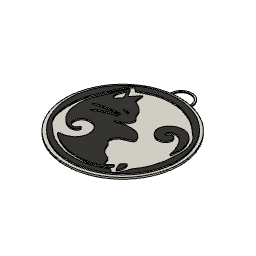
cats (Autodesk Fusion 360 design; units mm, degrees)
Autodesk Fusion 360 part; units mm, degrees
sketch "Sketch1" plane through (0, 0, 0) normal (0, 0, 1) x (1, 0, 0)
  spline S0 degree 3 poles (-11.5155, 73.2957) (-22.8925, 71.5759) (-32.7086, 67.8717) (-41.8102, 61.8657) knots 0 0 0 0 1 1 1 1
  spline S1 degree 3 poles (-41.8102, 61.8657) (-53.0815, 54.4309) (-62.9505, 42.6305) (-67.8452, 30.6977) knots 0 0 0 0 1 1 1 1
  spline S2 degree 3 poles (-67.8452, 30.6977) (-68.2421, 29.7452) (-68.7977, 28.4752) (-69.0623, 27.8667) knots 0 0 0 0 1 1 1 1
  spline S3 degree 3 poles (-69.0623, 27.8667) (-69.8561, 26.1469) (-71.9463, 18.9502) (-72.3696, 16.4632) knots 0 0 0 0 1 1 1 1
  spline S4 degree 3 poles (-72.3696, 16.4632) (-72.5813, 15.2461) (-72.8194, 14.1613) (-72.8723, 14.0555) knots 0 0 0 0 1 1 1 1
  spline S5 degree 3 poles (-72.8723, 14.0555) (-73.1634, 13.6057) (-73.8248, 4.5569) (-73.8248, 1.3025) knots 0 0 0 0 1 1 1 1
  spline S6 degree 3 poles (-73.8248, 1.3025) (-73.8248, -12.6939) (-69.1682, -26.955) (-60.4898, -39.4168) knots 0 0 0 0 1 1 1 1
  spline S7 degree 3 poles (-60.4898, -39.4168) (-58.4261, -42.4066) (-58.3732, -42.4595) (-54.96, -46.2431) knots 0 0 0 0 1 1 1 1
  spline S8 degree 3 poles (-54.96, -46.2431) (-51.0177, -50.6352) (-46.8373, -54.1541) (-41.2546, -57.8318) knots 0 0 0 0 1 1 1 1
  spline S9 degree 3 poles (-41.2546, -57.8318) (-37.8944, -60.0279) (-32.6292, -62.8325) (-29.3748, -64.1554) knots 0 0 0 0 1 1 1 1
  spline S10 degree 3 poles (-29.3748, -64.1554) (-28.4223, -64.5258) (-27.4169, -64.9491) (-27.1259, -65.0814) knots 0 0 0 0 1 1 1 1
  spline S11 degree 3 poles (-27.1259, -65.0814) (-25.9617, -65.5841) (-19.6117, -67.4627) (-18.0507, -67.7273) knots 0 0 0 0 1 1 1 1
  spline S12 degree 3 poles (-18.0507, -67.7273) (-17.1246, -67.886) (-16.0927, -68.1241) (-15.7752, -68.2564) knots 0 0 0 0 1 1 1 1
  spline S13 degree 3 poles (-15.7752, -68.2564) (-15.4577, -68.3623) (-13.7644, -68.6798) (-12.0182, -68.9708) knots 0 0 0 0 1 1 1 1
  spline S14 degree 3 poles (-12.0182, -68.9708) (-7.6261, -69.6323) (3.6716, -69.6323) (7.5345, -68.9443) knots 0 0 0 0 1 1 1 1
  spline S15 degree 3 poles (7.5345, -68.9443) (19.5202, -66.8277) (27.0873, -64.076) (35.7127, -58.7579) knots 0 0 0 0 1 1 1 1
  spline S16 degree 3 poles (35.7127, -58.7579) (48.201, -51.0056) (58.3081, -39.3375) (63.7585, -26.2935) knots 0 0 0 0 1 1 1 1
  spline S17 degree 3 poles (63.7585, -26.2935) (66.5631, -19.5995) (68.2035, -13.8052) (69.0502, -7.4023) knots 0 0 0 0 1 1 1 1
  spline S18 degree 3 poles (69.0502, -7.4023) (69.2089, -6.1587) (69.3941, -4.8623) (69.447, -4.4918) knots 0 0 0 0 1 1 1 1
  spline S19 degree 3 poles (69.447, -4.4918) (69.5264, -4.1214) (69.6323, -2.1106) (69.7381, 0.0061) knots 0 0 0 0 1 1 1 1
  spline S20 degree 3 poles (69.7381, 0.0061) (70.2143, 11.4096) (67.0923, 24.9298) (61.6154, 35.1427) knots 0 0 0 0 1 1 1 1
  spline S21 degree 3 poles (61.6154, 35.1427) (56.0327, 45.5673) (50.106, 52.5523) (40.8456, 59.6167) knots 0 0 0 0 1 1 1 1
  spline S22 degree 3 poles (40.8456, 59.6167) (31.3735, 66.8663) (19.0968, 71.814) (6.6614, 73.4015) knots 0 0 0 0 1 1 1 1
  spline S23 degree 3 poles (6.6614, 73.4015) (2.1106, 73.9836) (-7.2292, 73.9307) (-11.5155, 73.2957) knots 0 0 0 0 1 1 1 1
  spline S24 degree 3 poles (7.6668, 65.8609) (8.3283, 65.7286) (9.5718, 65.4905) (10.445, 65.3582) knots 0 0 0 0 1 1 1 1
  spline S25 degree 3 poles (10.445, 65.3582) (12.4293, 64.9877) (14.255, 64.4321) (20.2345, 62.2625) knots 0 0 0 0 1 1 1 1
  spline S26 degree 3 poles (20.2345, 62.2625) (26.1083, 60.1194) (28.0133, 59.2727) (31.982, 56.918) knots 0 0 0 0 1 1 1 1
  spline S27 degree 3 poles (31.982, 56.918) (36.427, 54.2986) (41.1631, 50.7002) (44.7085, 47.2607) knots 0 0 0 0 1 1 1 1
  spline S28 degree 3 poles (44.7085, 47.2607) (46.3754, 45.6467) (48.4656, 43.8475) (49.3387, 43.2655) knots 0 0 0 0 1 1 1 1
  spline S29 degree 3 poles (49.3387, 43.2655) (50.2118, 42.7098) (51.7993, 41.334) (52.8841, 40.2492) knots 0 0 0 0 1 1 1 1
  spline S30 degree 3 poles (52.8841, 40.2492) (54.8156, 38.2648) (58.4668, 33.423) (58.4668, 32.8409) knots 0 0 0 0 1 1 1 1
  spline S31 degree 3 poles (58.4668, 32.8409) (58.4668, 32.6821) (58.9431, 31.5973) (59.4987, 30.4596) knots 0 0 0 0 1 1 1 1
  spline S32 degree 3 poles (59.4987, 30.4596) (61.1391, 27.2052) (62.3033, 23.263) (62.9912, 18.6592) knots 0 0 0 0 1 1 1 1
  spline S33 degree 3 poles (62.9912, 18.6592) (63.3087, 16.3838) (63.15, 5.8798) (62.7002, 1.1173) knots 0 0 0 0 1 1 1 1
  spline S34 degree 3 poles (62.7002, 1.1173) (62.0387, -5.8148) (61.2714, -10.3656) (60.3454, -12.9585) knots 0 0 0 0 1 1 1 1
  spline S35 degree 3 poles (60.3454, -12.9585) (60.0014, -13.8845) (58.8373, -17.7475) (58.2287, -19.97) knots 0 0 0 0 1 1 1 1
  spline S36 degree 3 poles (58.2287, -19.97) (57.6202, -22.1925) (55.477, -27.0873) (54.1012, -29.4156) knots 0 0 0 0 1 1 1 1
  spline S37 degree 3 poles (54.1012, -29.4156) (53.5456, -30.3152) (52.0639, -32.617) (50.8468, -34.4691) knots 0 0 0 0 1 1 1 1
  spline S38 degree 3 poles (50.8468, -34.4691) (49.1006, -37.1414) (48.4656, -38.3585) (47.9893, -40.0254) knots 0 0 0 0 1 1 1 1
  spline S39 degree 3 poles (47.9893, -40.0254) (47.6454, -41.216) (47.3543, -42.3273) (47.3543, -42.5125) knots 0 0 0 0 1 1 1 1
  spline S40 degree 3 poles (47.3543, -42.5125) (47.3543, -43.1739) (45.2641, -47.6718) (44.2852, -49.1535) knots 0 0 0 0 1 1 1 1
  spline S41 degree 3 poles (44.2852, -49.1535) (41.9568, -52.6195) (40.8456, -53.8102) (39.5491, -54.3129) knots 0 0 0 0 1 1 1 1
  spline S42 degree 3 poles (39.5491, -54.3129) (38.0939, -54.842) (37.8823, -54.7362) (36.9827, -53.1223) knots 0 0 0 0 1 1 1 1
  spline S43 degree 3 poles (36.9827, -53.1223) (36.4006, -52.1168) (35.3687, -51.3231) (34.575, -51.3231) knots 0 0 0 0 1 1 1 1
  spline S44 degree 3 poles (34.575, -51.3231) (34.3898, -51.3231) (32.9345, -52.1698) (31.3206, -53.2281) knots 0 0 0 0 1 1 1 1
  spline S45 degree 3 poles (31.3206, -53.2281) (28.3043, -55.2125) (24.5737, -57.0645) (22.3512, -57.7525) knots 0 0 0 0 1 1 1 1
  spline S46 degree 3 poles (22.3512, -57.7525) (21.6368, -57.9641) (20.1023, -58.5198) (18.9645, -58.9695) knots 0 0 0 0 1 1 1 1
  spline S47 degree 3 poles (18.9645, -58.9695) (17.8268, -59.4193) (16.4775, -59.8956) (15.9218, -60.0279) knots 0 0 0 0 1 1 1 1
  spline S48 degree 3 poles (15.9218, -60.0279) (15.3927, -60.1602) (13.7523, -60.5835) (12.297, -60.9275) knots 0 0 0 0 1 1 1 1
  spline S49 degree 3 poles (12.297, -60.9275) (10.8418, -61.2979) (8.0373, -61.8535) (6.0793, -62.1975) knots 0 0 0 0 1 1 1 1
  spline S50 degree 3 poles (6.0793, -62.1975) (2.825, -62.7266) (1.9783, -62.7531) (-3.7102, -62.5943) knots 0 0 0 0 1 1 1 1
  spline S51 degree 3 poles (-3.7102, -62.5943) (-9.4517, -62.4356) (-13.8438, -62.0123) (-16.1457, -61.4037) knots 0 0 0 0 1 1 1 1
  spline S52 degree 3 poles (-16.1457, -61.4037) (-16.6484, -61.2714) (-17.7332, -60.9539) (-18.5269, -60.7158) knots 0 0 0 0 1 1 1 1
  spline S53 degree 3 poles (-18.5269, -60.7158) (-19.3207, -60.4777) (-21.0405, -60.0014) (-22.3634, -59.6575) knots 0 0 0 0 1 1 1 1
  spline S54 degree 3 poles (-22.3634, -59.6575) (-30.5655, -57.4614) (-40.7784, -51.9581) (-46.3082, -46.6929) knots 0 0 0 0 1 1 1 1
  spline S55 degree 3 poles (-46.3082, -46.6929) (-47.5517, -45.5287) (-49.9859, -43.412) (-51.7321, -42.0098) knots 0 0 0 0 1 1 1 1
  spline S56 degree 3 poles (-51.7321, -42.0098) (-55.0659, -39.3639) (-57.0502, -37.4589) (-58.5584, -35.4481) knots 0 0 0 0 1 1 1 1
  spline S57 degree 3 poles (-58.5584, -35.4481) (-59.9607, -33.596) (-62.8975, -28.2779) (-63.4796, -26.5581) knots 0 0 0 0 1 1 1 1
  spline S58 degree 3 poles (-63.4796, -26.5581) (-64.8025, -22.5629) (-65.8873, -17.7739) (-65.8873, -15.9748) knots 0 0 0 0 1 1 1 1
  spline S59 degree 3 poles (-65.8873, -15.9748) (-65.8873, -15.3398) (-66.0725, -13.9639) (-66.3107, -12.9056) knots 0 0 0 0 1 1 1 1
  spline S60 degree 3 poles (-66.3107, -12.9056) (-66.6546, -11.2916) (-66.7075, -9.8629) (-66.5752, -4.095) knots 0 0 0 0 1 1 1 1
  spline S61 degree 3 poles (-66.5752, -4.095) (-66.39, 3.1546) (-66.1255, 6.3825) (-65.5169, 8.9225) knots 0 0 0 0 1 1 1 1
  spline S62 degree 3 poles (-65.5169, 8.9225) (-65.3052, 9.7692) (-64.8819, 11.6477) (-64.5644, 13.103) knots 0 0 0 0 1 1 1 1
  spline S63 degree 3 poles (-64.5644, 13.103) (-64.2734, 14.5582) (-63.8765, 16.278) (-63.7177, 16.9394) knots 0 0 0 0 1 1 1 1
  spline S64 degree 3 poles (-63.7177, 16.9394) (-63.1886, 19.1619) (-58.9552, 29.5071) (-57.4471, 32.2852) knots 0 0 0 0 1 1 1 1
  spline S65 degree 3 poles (-57.4471, 32.2852) (-56.6005, 33.8198) (-55.7802, 35.619) (-55.6215, 36.3334) knots 0 0 0 0 1 1 1 1
  spline S66 degree 3 poles (-55.6215, 36.3334) (-55.4363, 37.0213) (-54.9865, 38.2648) (-54.6161, 39.1115) knots 0 0 0 0 1 1 1 1
  spline S67 degree 3 poles (-54.6161, 39.1115) (-54.2457, 39.9317) (-53.6371, 41.4663) (-53.2667, 42.4717) knots 0 0 0 0 1 1 1 1
  spline S68 degree 3 poles (-53.2667, 42.4717) (-52.473, 44.6942) (-49.3773, 51.1236) (-47.6046, 54.2457) knots 0 0 0 0 1 1 1 1
  spline S69 degree 3 poles (-47.6046, 54.2457) (-46.9167, 55.4892) (-45.7525, 57.0767) (-45.0117, 57.7911) knots 0 0 0 0 1 1 1 1
  line L0 (-45.0117, 57.7911) -> (-43.7152, 59.0875)
  line L1 (-43.7152, 59.0875) -> (-42.6834, 58.4525)
  spline S70 degree 3 poles (-42.6834, 58.4525) (-42.1277, 58.1086) (-41.043, 57.2619) (-40.3021, 56.5475) knots 0 0 0 0 1 1 1 1
  spline S71 degree 3 poles (-40.3021, 56.5475) (-39.0321, 55.3569) (-38.8205, 55.2511) (-37.9473, 55.3834) knots 0 0 0 0 1 1 1 1
  spline S72 degree 3 poles (-37.9473, 55.3834) (-37.4182, 55.4627) (-35.3015, 56.4946) (-33.2642, 57.6588) knots 0 0 0 0 1 1 1 1
  spline S73 degree 3 poles (-33.2642, 57.6588) (-31.2005, 58.823) (-28.978, 60.0136) (-28.3165, 60.3046) knots 0 0 0 0 1 1 1 1
  spline S74 degree 3 poles (-28.3165, 60.3046) (-22.0459, 63.0827) (-19.8498, 64.0352) (-19.5852, 64.0352) knots 0 0 0 0 1 1 1 1
  spline S75 degree 3 poles (-19.5852, 64.0352) (-19.4, 64.0352) (-18.2888, 64.2469) (-17.0982, 64.538) knots 0 0 0 0 1 1 1 1
  spline S76 degree 3 poles (-17.0982, 64.538) (-13.4734, 65.3846) (-10.2719, 65.9138) (-7.388, 66.1519) knots 0 0 0 0 1 1 1 1
  spline S77 degree 3 poles (-7.388, 66.1519) (-4.16, 66.4165) (5.947, 66.2313) (7.6668, 65.8609) knots 0 0 0 0 1 1 1 1
  spline S78 degree 3 poles (-29.6394, 52.0496) (-30.5919, 50.859) (-32.0207, 48.9805) (-32.8409, 47.8957) knots 0 0 0 0 1 1 1 1
  spline S79 degree 3 poles (-32.8409, 47.8957) (-33.6611, 46.8109) (-34.7459, 45.5144) (-35.2486, 45.0382) knots 0 0 0 0 1 1 1 1
  line L2 (-35.2486, 45.0382) -> (-36.2011, 44.1386)
  line L3 (-36.2011, 44.1386) -> (-37.3388, 44.5355)
  spline S80 degree 3 poles (-37.3388, 44.5355) (-38.3707, 44.8794) (-38.6617, 45.1705) (-39.773, 46.9961) knots 0 0 0 0 1 1 1 1
  spline S81 degree 3 poles (-39.773, 46.9961) (-40.4609, 48.1602) (-41.4663, 49.9594) (-42.0219, 51.0177) knots 0 0 0 0 1 1 1 1
  spline S82 degree 3 poles (-42.0219, 51.0177) (-43.3184, 53.5313) (-44.0857, 53.7959) (-45.0911, 52.0496) knots 0 0 0 0 1 1 1 1
  spline S83 degree 3 poles (-45.0911, 52.0496) (-45.9377, 50.568) (-47.8163, 46.7315) (-48.028, 46.0436) knots 0 0 0 0 1 1 1 1
  spline S84 degree 3 poles (-48.028, 46.0436) (-48.2132, 45.3821) (-48.7423, 44.165) (-49.88, 41.678) knots 0 0 0 0 1 1 1 1
  spline S85 degree 3 poles (-49.88, 41.678) (-50.4886, 40.3286) (-51.0971, 38.5294) (-52.129, 34.9311) knots 0 0 0 0 1 1 1 1
  spline S86 degree 3 poles (-52.129, 34.9311) (-52.4465, 33.8463) (-53.69, 30.9094) (-54.9071, 28.4488) knots 0 0 0 0 1 1 1 1
  spline S87 degree 3 poles (-54.9071, 28.4488) (-60.4369, 17.1775) (-62.2096, 9.3194) (-61.4688, -0.576) knots 0 0 0 0 1 1 1 1
  spline S88 degree 3 poles (-61.4688, -0.576) (-60.7015, -10.5243) (-57.8705, -17.8004) (-52.6846, -22.9598) knots 0 0 0 0 1 1 1 1
  spline S89 degree 3 poles (-52.6846, -22.9598) (-47.2871, -28.3573) (-43.8475, -30.1035) (-39.0586, -29.8125) knots 0 0 0 0 1 1 1 1
  spline S90 degree 3 poles (-39.0586, -29.8125) (-35.8042, -29.6273) (-34.349, -29.0452) (-33.0525, -27.4048) knots 0 0 0 0 1 1 1 1
  spline S91 degree 3 poles (-33.0525, -27.4048) (-31.8884, -25.976) (-31.6767, -25.3675) (-31.809, -24.0445) knots 0 0 0 0 1 1 1 1
  spline S92 degree 3 poles (-31.809, -24.0445) (-31.8619, -23.3831) (-32.1, -23.0391) (-32.735, -22.6952) knots 0 0 0 0 1 1 1 1
  line L4 (-32.735, -22.6952) -> (-33.5552, -22.1925)
  line L5 (-33.5552, -22.1925) -> (-35.0634, -24.2562)
  spline S93 degree 3 poles (-35.0634, -24.2562) (-36.9155, -26.7962) (-37.0477, -26.902) (-38.6088, -27.1137) knots 0 0 0 0 1 1 1 1
  spline S94 degree 3 poles (-38.6088, -27.1137) (-40.4873, -27.3783) (-42.4717, -26.4258) (-43.7682, -24.6266) knots 0 0 0 0 1 1 1 1
  spline S95 degree 3 poles (-43.7682, -24.6266) (-44.7207, -23.3302) (-44.7736, -23.1714) (-44.9059, -20.6579) knots 0 0 0 0 1 1 1 1
  spline S96 degree 3 poles (-44.9059, -20.6579) (-45.0911, -17.6152) (-44.7207, -16.1864) (-43.2919, -13.9375) knots 0 0 0 0 1 1 1 1
  spline S97 degree 3 poles (-43.2919, -13.9375) (-41.7838, -11.6356) (-40.5402, -10.8418) (-37.3123, -10.1539) knots 0 0 0 0 1 1 1 1
  spline S98 degree 3 poles (-37.3123, -10.1539) (-34.693, -9.6248) (-32.8673, -9.6248) (-30.4067, -10.1804) knots 0 0 0 0 1 1 1 1
  spline S99 degree 3 poles (-30.4067, -10.1804) (-27.655, -10.7889) (-26.2792, -11.5033) (-24.6388, -13.1437) knots 0 0 0 0 1 1 1 1
  spline S100 degree 3 poles (-24.6388, -13.1437) (-22.8132, -14.9958) (-21.8871, -16.5833) (-20.8817, -19.626) knots 0 0 0 0 1 1 1 1
  spline S101 degree 3 poles (-20.8817, -19.626) (-20.2202, -21.6368) (-20.1144, -22.3512) (-20.1144, -24.9177) knots 0 0 0 0 1 1 1 1
  spline S102 degree 3 poles (-20.1144, -24.9177) (-20.1144, -29.6537) (-21.1727, -32.4583) (-24.5859, -36.771) knots 0 0 0 0 1 1 1 1
  spline S103 degree 3 poles (-24.5859, -36.771) (-26.4644, -39.1523) (-27.5757, -39.9195) (-32.153, -42.0098) knots 0 0 0 0 1 1 1 1
  spline S104 degree 3 poles (-32.153, -42.0098) (-34.9311, -43.2798) (-35.2221, -43.3591) (-38.5823, -43.6766) knots 0 0 0 0 1 1 1 1
  spline S105 degree 3 poles (-38.5823, -43.6766) (-42.3923, -44.0206) (-42.3923, -44.0206) (-41.2017, -45.4758) knots 0 0 0 0 1 1 1 1
  spline S106 degree 3 poles (-41.2017, -45.4758) (-40.4609, -46.4283) (-34.058, -50.6881) (-31.5444, -51.9581) knots 0 0 0 0 1 1 1 1
  spline S107 degree 3 poles (-31.5444, -51.9581) (-29.0044, -53.2281) (-25.5384, -54.6568) (-22.9455, -55.4506) knots 0 0 0 0 1 1 1 1
  spline S108 degree 3 poles (-22.9455, -55.4506) (-21.8342, -55.7945) (-19.9292, -56.4031) (-18.7121, -56.7735) knots 0 0 0 0 1 1 1 1
  spline S109 degree 3 poles (-18.7121, -56.7735) (-13.3411, -58.4404) (-4.6363, -59.2341) (2.481, -58.7579) knots 0 0 0 0 1 1 1 1
  spline S110 degree 3 poles (2.481, -58.7579) (8.1166, -58.361) (11.3181, -57.7525) (15.7366, -56.2443) knots 0 0 0 0 1 1 1 1
  spline S111 degree 3 poles (15.7366, -56.2443) (22.2189, -54.0218) (25.8437, -52.355) (29.786, -49.7091) knots 0 0 0 0 1 1 1 1
  spline S112 degree 3 poles (29.786, -49.7091) (31.7968, -48.3598) (32.326, -47.8041) (33.1991, -46.2166) knots 0 0 0 0 1 1 1 1
  line L6 (33.1991, -46.2166) -> (33.7283, -45.2377)
  line L7 (33.7283, -45.2377) -> (32.9875, -44.5233)
  spline S113 degree 3 poles (32.9875, -44.5233) (32.4318, -43.9412) (32.1937, -43.8618) (32.035, -44.1264) knots 0 0 0 0 1 1 1 1
  spline S114 degree 3 poles (32.035, -44.1264) (31.9291, -44.3381) (30.8179, -45.5023) (29.6008, -46.7458) knots 0 0 0 0 1 1 1 1
  spline S115 degree 3 poles (29.6008, -46.7458) (27.3783, -48.9948) (25.6585, -50.1589) (24.9706, -49.8943) knots 0 0 0 0 1 1 1 1
  spline S116 degree 3 poles (24.9706, -49.8943) (24.3885, -49.6827) (23.6477, -47.9364) (22.9068, -44.9731) knots 0 0 0 0 1 1 1 1
  spline S117 degree 3 poles (22.9068, -44.9731) (22.0602, -41.7187) (21.3987, -40.8456) (19.0704, -39.9195) knots 0 0 0 0 1 1 1 1
  spline S118 degree 3 poles (19.0704, -39.9195) (15.0223, -38.332) (12.8791, -36.9827) (10.445, -34.5485) knots 0 0 0 0 1 1 1 1
  spline S119 degree 3 poles (10.445, -34.5485) (7.905, -31.982) (6.5291, -29.7595) (5.7089, -26.9814) knots 0 0 0 0 1 1 1 1
  spline S120 degree 3 poles (5.7089, -26.9814) (5.2062, -25.2352) (3.7775, -23.2508) (1.9518, -21.7691) knots 0 0 0 0 1 1 1 1
  spline S121 degree 3 poles (1.9518, -21.7691) (0.7348, -20.7902) (0.576, -20.5256) (0.4173, -19.335) knots 0 0 0 0 1 1 1 1
  spline S122 degree 3 poles (0.4173, -19.335) (0.1262, -17.0331) (1.1581, -14.1756) (3.3806, -11.2387) knots 0 0 0 0 1 1 1 1
  spline S123 degree 3 poles (3.3806, -11.2387) (4.5448, -9.7041) (5.4708, -9.122) (9.2543, -7.6404) knots 0 0 0 0 1 1 1 1
  spline S124 degree 3 poles (9.2543, -7.6404) (12.7998, -6.2381) (16.1864, -4.5712) (17.2183, -3.6981) knots 0 0 0 0 1 1 1 1
  spline S125 degree 3 poles (17.2183, -3.6981) (19.0968, -2.137) (18.1179, 1.4613) (14.9693, 4.6363) knots 0 0 0 0 1 1 1 1
  spline S126 degree 3 poles (14.9693, 4.6363) (12.2706, 7.335) (8.6987, 8.7373) (3.1689, 9.293) knots 0 0 0 0 1 1 1 1
  spline S127 degree 3 poles (3.1689, 9.293) (0.8141, 9.5311) (-0.6411, 9.5311) (-2.7048, 9.293) knots 0 0 0 0 1 1 1 1
  spline S128 degree 3 poles (-2.7048, 9.293) (-5.7211, 8.9755) (-6.9646, 8.6315) (-12.9177, 6.4355) knots 0 0 0 0 1 1 1 1
  spline S129 degree 3 poles (-12.9177, 6.4355) (-15.299, 5.5623) (-17.0452, 5.0596) (-17.1775, 5.1919) knots 0 0 0 0 1 1 1 1
  spline S130 degree 3 poles (-17.1775, 5.1919) (-17.3098, 5.3242) (-17.3627, 5.8005) (-17.2834, 6.2767) knots 0 0 0 0 1 1 1 1
  spline S131 degree 3 poles (-17.2834, 6.2767) (-17.0982, 7.388) (-15.2196, 8.6315) (-11.9123, 9.7957) knots 0 0 0 0 1 1 1 1
  spline S132 degree 3 poles (-11.9123, 9.7957) (-8.6844, 10.9334) (-7.4938, 12.0975) (-5.5888, 15.9605) knots 0 0 0 0 1 1 1 1
  spline S133 degree 3 poles (-5.5888, 15.9605) (-3.4192, 20.3261) (-3.6044, 21.2786) (-7.1763, 24.4007) knots 0 0 0 0 1 1 1 1
  spline S134 degree 3 poles (-7.1763, 24.4007) (-8.8961, 25.9088) (-9.584, 27.02) (-10.3248, 29.56) knots 0 0 0 0 1 1 1 1
  spline S135 degree 3 poles (-10.3248, 29.56) (-11.0127, 31.8884) (-11.9123, 33.2377) (-14.2142, 35.4867) knots 0 0 0 0 1 1 1 1
  spline S136 degree 3 poles (-14.2142, 35.4867) (-17.0982, 38.2648) (-17.7596, 38.7146) (-21.3844, 40.3286) knots 0 0 0 0 1 1 1 1
  spline S137 degree 3 poles (-21.3844, 40.3286) (-23.1571, 41.1223) (-24.9298, 41.9955) (-25.3267, 42.2865) knots 0 0 0 0 1 1 1 1
  spline S138 degree 3 poles (-25.3267, 42.2865) (-26.6232, 43.2125) (-27.1788, 45.3292) (-27.364, 49.88) knots 0 0 0 0 1 1 1 1
  spline S139 degree 3 poles (-27.364, 49.88) (-27.4698, 52.0496) (-27.6286, 53.9282) (-27.7344, 54.034) knots 0 0 0 0 1 1 1 1
  spline S140 degree 3 poles (-27.7344, 54.034) (-27.8402, 54.1398) (-28.7134, 53.2402) (-29.6394, 52.0496) knots 0 0 0 0 1 1 1 1
  spline S141 degree 3 poles (-42.8157, 47.3136) (-42.313, 46.6786) (-41.2282, 45.0382) (-40.408, 43.6359) knots 0 0 0 0 1 1 1 1
  spline S142 degree 3 poles (-40.408, 43.6359) (-39.0057, 41.2811) (-38.8998, 40.99) (-38.8998, 39.4555) knots 0 0 0 0 1 1 1 1
  spline S143 degree 3 poles (-38.8998, 39.4555) (-38.8998, 37.815) (-38.9263, 37.7621) (-40.1434, 36.545) knots 0 0 0 0 1 1 1 1
  spline S144 degree 3 poles (-40.1434, 36.545) (-40.8577, 35.8836) (-41.8102, 34.7459) (-42.26, 34.058) knots 0 0 0 0 1 1 1 1
  spline S145 degree 3 poles (-42.26, 34.058) (-43.7946, 31.8355) (-45.435, 31.7032) (-46.6786, 33.6875) knots 0 0 0 0 1 1 1 1
  spline S146 degree 3 poles (-46.6786, 33.6875) (-47.3665, 34.7988) (-47.4723, 35.275) (-47.5782, 37.2594) knots 0 0 0 0 1 1 1 1
  spline S147 degree 3 poles (-47.5782, 37.2594) (-47.684, 39.5084) (-47.6311, 39.6407) (-46.2288, 43.4242) knots 0 0 0 0 1 1 1 1
  spline S148 degree 3 poles (-46.2288, 43.4242) (-44.6677, 47.6046) (-44.2973, 48.4248) (-43.9534, 48.4248) knots 0 0 0 0 1 1 1 1
  spline S149 degree 3 poles (-43.9534, 48.4248) (-43.8211, 48.4248) (-43.3184, 47.9221) (-42.8157, 47.3136) knots 0 0 0 0 1 1 1 1
  spline S150 degree 3 poles (-17.7596, 25.9088) (-17.0188, 25.6442) (-16.9394, 25.5119) (-16.9394, 24.5065) knots 0 0 0 0 1 1 1 1
  spline S151 degree 3 poles (-16.9394, 24.5065) (-16.9394, 23.8715) (-16.9923, 23.3159) (-17.0982, 23.2365) knots 0 0 0 0 1 1 1 1
  spline S152 degree 3 poles (-17.0982, 23.2365) (-17.1775, 23.1571) (-17.7861, 23.263) (-18.474, 23.4746) knots 0 0 0 0 1 1 1 1
  spline S153 degree 3 poles (-18.474, 23.4746) (-19.1619, 23.6863) (-20.4319, 24.0302) (-21.305, 24.2419) knots 0 0 0 0 1 1 1 1
  spline S154 degree 3 poles (-21.305, 24.2419) (-23.5275, 24.7711) (-24.6123, 25.1415) (-24.6123, 25.3796) knots 0 0 0 0 1 1 1 1
  spline S155 degree 3 poles (-24.6123, 25.3796) (-24.6123, 26.0146) (-19.2677, 26.438) (-17.7596, 25.9088) knots 0 0 0 0 1 1 1 1
  spline S156 degree 3 poles (-21.7548, 18.5005) (-20.1938, 17.9184) (-22.1252, 17.0717) (-26.1469, 16.5425) knots 0 0 0 0 1 1 1 1
  spline S157 degree 3 poles (-26.1469, 16.5425) (-29.6394, 16.1192) (-31.2269, 15.8282) (-37.8415, 14.4788) knots 0 0 0 0 1 1 1 1
  spline S158 degree 3 poles (-37.8415, 14.4788) (-42.604, 13.4998) (-45.9907, 12.6002) (-48.4777, 11.6477) knots 0 0 0 0 1 1 1 1
  spline S159 degree 3 poles (-48.4777, 11.6477) (-49.9065, 11.1186) (-50.9913, 10.9863) (-52.0496, 11.2773) knots 0 0 0 0 1 1 1 1
  spline S160 degree 3 poles (-52.0496, 11.2773) (-52.8698, 11.5155) (-52.8169, 11.78) (-51.7321, 12.6002) knots 0 0 0 0 1 1 1 1
  spline S161 degree 3 poles (-51.7321, 12.6002) (-50.1182, 13.8438) (-44.7736, 15.3784) (-37.3123, 16.8071) knots 0 0 0 0 1 1 1 1
  spline S162 degree 3 poles (-37.3123, 16.8071) (-36.2275, 17.0188) (-34.1373, 17.4421) (-32.6821, 17.7596) knots 0 0 0 0 1 1 1 1
  spline S163 degree 3 poles (-32.6821, 17.7596) (-27.4698, 18.8709) (-23.4746, 19.1355) (-21.7548, 18.5005) knots 0 0 0 0 1 1 1 1
  spline S164 degree 3 poles (-20.8552, 15.2461) (-20.4055, 14.2142) (-20.6965, 13.9232) (-22.7867, 13.394) knots 0 0 0 0 1 1 1 1
  spline S165 degree 3 poles (-22.7867, 13.394) (-29.269, 11.7536) (-35.6455, 8.949) (-42.1807, 4.848) knots 0 0 0 0 1 1 1 1
  spline S166 degree 3 poles (-42.1807, 4.848) (-44.0327, 3.6838) (-45.1175, 3.1811) (-45.6996, 3.1811) knots 0 0 0 0 1 1 1 1
  spline S167 degree 3 poles (-45.6996, 3.1811) (-46.9167, 3.1811) (-46.8109, 3.6838) (-45.2763, 5.1125) knots 0 0 0 0 1 1 1 1
  spline S168 degree 3 poles (-45.2763, 5.1125) (-41.3869, 8.7638) (-32.2059, 13.0765) (-23.0248, 15.59) knots 0 0 0 0 1 1 1 1
  spline S169 degree 3 poles (-23.0248, 15.59) (-21.5432, 15.9869) (-21.1727, 15.934) (-20.8552, 15.2461) knots 0 0 0 0 1 1 1 1
  spline S170 degree 3 poles (33.1991, 41.5721) (29.3362, 40.4873) (27.7223, 39.5613) (24.6002, 36.598) knots 0 0 0 0 1 1 1 1
  spline S171 degree 3 poles (24.6002, 36.598) (23.0127, 35.1163) (22.6423, 34.5871) (21.5575, 32.0736) knots 0 0 0 0 1 1 1 1
  spline S172 degree 3 poles (21.5575, 32.0736) (20.4462, 29.56) (20.2875, 28.978) (20.1552, 26.8348) knots 0 0 0 0 1 1 1 1
  spline S173 degree 3 poles (20.1552, 26.8348) (20.0229, 24.2684) (20.3139, 23.0513) (21.7956, 20.1673) knots 0 0 0 0 1 1 1 1
  spline S174 degree 3 poles (21.7956, 20.1673) (23.436, 16.9923) (28.3573, 14.0025) (31.982, 14.029) knots 0 0 0 0 1 1 1 1
  spline S175 degree 3 poles (31.982, 14.029) (34.9983, 14.0555) (37.9087, 15.0873) (39.6285, 16.7542) knots 0 0 0 0 1 1 1 1
  spline S176 degree 3 poles (39.6285, 16.7542) (41.0573, 18.13) (41.9039, 19.744) (42.2743, 21.8342) knots 0 0 0 0 1 1 1 1
  spline S177 degree 3 poles (42.2743, 21.8342) (42.5389, 23.21) (42.5125, 23.6069) (42.0891, 24.824) knots 0 0 0 0 1 1 1 1
  spline S178 degree 3 poles (42.0891, 24.824) (41.4541, 26.6761) (39.6814, 28.0519) (37.9087, 28.0519) knots 0 0 0 0 1 1 1 1
  spline S179 degree 3 poles (37.9087, 28.0519) (36.2154, 28.0519) (34.8131, 27.0465) (34.231, 25.3796) knots 0 0 0 0 1 1 1 1
  line L8 (34.231, 25.3796) -> (33.7548, 24.0567)
  line L9 (33.7548, 24.0567) -> (32.5377, 24.2419)
  spline S180 degree 3 poles (32.5377, 24.2419) (31.8762, 24.3213) (31.2412, 24.5065) (31.1089, 24.6388) knots 0 0 0 0 1 1 1 1
  spline S181 degree 3 poles (31.1089, 24.6388) (30.9766, 24.7446) (30.8179, 25.4855) (30.7385, 26.2792) knots 0 0 0 0 1 1 1 1
  spline S182 degree 3 poles (30.7385, 26.2792) (30.6327, 27.5757) (30.712, 27.8138) (31.5852, 29.0309) knots 0 0 0 0 1 1 1 1
  spline S183 degree 3 poles (31.5852, 29.0309) (33.4902, 31.7032) (37.8558, 32.7615) (41.5864, 31.465) knots 0 0 0 0 1 1 1 1
  spline S184 degree 3 poles (41.5864, 31.465) (45.37, 30.1686) (49.9473, 25.2473) (52.7518, 19.4794) knots 0 0 0 0 1 1 1 1
  spline S185 degree 3 poles (52.7518, 19.4794) (56.2973, 12.2034) (56.747, 10.9598) (56.9852, 7.8113) knots 0 0 0 0 1 1 1 1
  spline S186 degree 3 poles (56.9852, 7.8113) (57.1968, 5.483) (57.382, 4.7686) (57.8318, 4.7686) knots 0 0 0 0 1 1 1 1
  spline S187 degree 3 poles (57.8318, 4.7686) (58.6256, 4.7686) (59.34, 9.3459) (59.34, 14.4259) knots 0 0 0 0 1 1 1 1
  spline S188 degree 3 poles (59.34, 14.4259) (59.34, 18.13) (59.2606, 19.0296) (58.6256, 21.5696) knots 0 0 0 0 1 1 1 1
  spline S189 degree 3 poles (58.6256, 21.5696) (57.8848, 24.6652) (57.8583, 24.7711) (56.747, 27.655) knots 0 0 0 0 1 1 1 1
  spline S190 degree 3 poles (56.747, 27.655) (54.6304, 33.1584) (52.3285, 36.0688) (47.7777, 39.138) knots 0 0 0 0 1 1 1 1
  spline S191 degree 3 poles (47.7777, 39.138) (46.64, 39.9317) (44.8937, 40.9107) (43.9412, 41.334) knots 0 0 0 0 1 1 1 1
  spline S192 degree 3 poles (43.9412, 41.334) (42.3802, 42.0484) (41.8775, 42.1542) (39.02, 42.2336) knots 0 0 0 0 1 1 1 1
  spline S193 degree 3 poles (39.02, 42.2336) (36.1625, 42.313) (35.5804, 42.26) (33.1991, 41.5721) knots 0 0 0 0 1 1 1 1
  spline S194 degree 3 poles (37.697, -36.8239) (35.7391, -38.9406) (35.6862, -39.0729) (35.792, -40.1048) knots 0 0 0 0 1 1 1 1
  spline S195 degree 3 poles (35.792, -40.1048) (35.9508, -41.6658) (38.0145, -46.8781) (38.8083, -47.7248) knots 0 0 0 0 1 1 1 1
  line L10 (38.8083, -47.7248) -> (39.4433, -48.4391)
  line L11 (39.4433, -48.4391) -> (40.1312, -47.4337)
  spline S196 degree 3 poles (40.1312, -47.4337) (41.2954, -45.7404) (42.3008, -43.3856) (42.4595, -41.9568) knots 0 0 0 0 1 1 1 1
  spline S197 degree 3 poles (42.4595, -41.9568) (42.6183, -40.581) (42.142, -37.8029) (41.4012, -36.0831) knots 0 0 0 0 1 1 1 1
  spline S198 degree 3 poles (41.4012, -36.0831) (41.1102, -35.3687) (40.3429, -34.6543) (39.8666, -34.6543) knots 0 0 0 0 1 1 1 1
  spline S199 degree 3 poles (39.8666, -34.6543) (39.7873, -34.6543) (38.8083, -35.6333) (37.697, -36.8239) knots 0 0 0 0 1 1 1 1
extrude "Extrude1" add sketch "Sketch1" along normal blind 2 makes body 1 at (-0.7491, 68.6059, 0) makes body 2 at (38.4886, -42.736, 0) makes body 3 at (-6.853, -41.4562, 0) makes body 4 at (55.9568, 16.8566, 0)
sketch "Sketch2" plane through (0, 0, 0) normal (0, 0, 1) x (1, 0, 0)
  circle A0 centre (-2.2405, 1.8984) radius 75.7684
extrude "Extrude2" add sketch "Sketch2" along normal mid plane 1 bodies 1 2 3 4
extrude "Extrude3" add 1 faces at (18.6271, -12.3289, -0.5) along direction (0, 0, -1) blind 1 on bodies 1 bodies 1
sketch "Sketch3" plane through (0, 0, 0) normal (0, 0, 1) x (1, 0, 0)
  circle A0 centre (0, 77.305) radius 12.5
  circle A1 centre (0, 77.305) radius 14.5
  dimension "d7" = 25
  dimension "d8" = 2
  measures "d7" diameter of A0
extrude "Extrude4" add sketch "Sketch3" against normal blind 1 bodies 1
